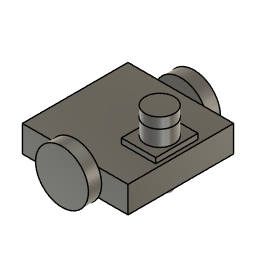
ros2bot (Autodesk Fusion 360 design; units mm, degrees)
Autodesk Fusion 360 part; units mm, degrees
sketch "Sketch1" plane through (0, 0, 0) normal (0, 0, 1) x (1, 0, 0)
  line L0 (-100, -100) -> (100, -100)
  line L1 (100, -100) -> (100, 100)
  line L2 (100, 100) -> (-100, 100)
  line L3 (-100, 100) -> (-100, -100)
  line L4 (-100, -100) -> (100, 100) construction
  line L5 (100, -100) -> (-100, 100) construction
  dimension "d1" = 200
  constraint horizontal L0
  constraint perpendicular L0 L1
  constraint parallel L0 L2
  constraint parallel L1 L3
  constraint coincident L4 origin
  constraint coincident L5 origin
  measures "d1" distance of L0.end L1.end
extrude "Extrude1" add sketch "Sketch1" along normal blind 50 makes body 1
sketch "Sketch2" plane through (0, -100, 0) normal (0, -1, 0) x (1, 0, 0)
  line L0 (-100, 0) -> (100, 0)
  line L1 (100, 0) -> (100, 50)
  line L2 (100, 50) -> (-100, 50)
  line L3 (-100, 50) -> (-100, 0)
  circle A0 centre (0, 25) radius 50
  dimension "d4" = 100
  measures "d4" diameter of A0
extrude "Extrude2" add sketch "Sketch2" along normal blind 25 separate body contours L0 L2 A0 | L0 A0 | L2 A0 makes body 2
mirror "Mirror1" about plane through (0, 0, 0) normal (0, 1, 0) of bodies 2 makes body 3
ref_plane "WorkPlane1" through (0, -116.4058, -25) normal (0, 0, -1) x (-1, 0, 0)
move_body "Move1" bodies 3 2 1 to x (1, 0, 0) y (0, 1, 0) z (0, 0, 1) at (0, 0, 25)
sketch "Sketch3" plane through (0, 0, 25) normal (0, 0, -1) x (1, 0, 0)
  line L0 (-100, 100) -> (-100, -100)
  line L1 (-100, -100) -> (100, -100)
  line L2 (100, -100) -> (100, 100)
  line L3 (100, 100) -> (-100, 100)
  circle A0 centre (75, 0) radius 10
  circle A1 centre (-70, 0) radius 10
  dimension "d10" = 20
  dimension "d11" = 20
  measures "d10" diameter of A0
  measures "d11" diameter of A1
extrude "Extrude3" add sketch "Sketch3" along normal blind 25 contours A0 | A1 bodies 1
fillet "Fillet1" radius 10 2 faces at (-70.8877, -1.6566, 0) (72.4279, -1.414, 0) on bodies 1
sketch "Sketch4" plane through (0, 0, 75) normal (0, 0, 1) x (-1, 0, 0)
  line L0 (100, -100) -> (100, 100)
  line L1 (100, 100) -> (-100, 100)
  line L2 (-100, 100) -> (-100, -100)
  line L3 (-100, -100) -> (100, -100)
  line L4 (-27.5, 40) -> (-92.5, 40)
  line L5 (-92.5, 40) -> (-92.5, -40)
  line L6 (-92.5, -40) -> (-27.5, -40)
  line L7 (-27.5, -40) -> (-27.5, 40)
  line L8 (-27.5, 40) -> (-92.5, -40) construction
  line L9 (-92.5, 40) -> (-27.5, -40) construction
  point P0 (-60, 0)
  dimension "d16" = 65
  dimension "d17" = 80
  constraint horizontal L4
  constraint perpendicular L4 L5
  constraint parallel L4 L6
  constraint parallel L5 L7
  constraint coincident L8 P0
  constraint coincident L9 P0
  measures "d16" distance of L5.end L6.end
  measures "d17" distance of L4.end L5.end
extrude "Extrude4" add sketch "Sketch4" along normal blind 10 contours L4 L5 L6 L7 bodies 1
sketch "Sketch5" plane through (0, 0, 85) normal (0, 0, 1) x (-1, 0, 0)
  line L0 (-27.5, -40) -> (-27.5, 40)
  line L1 (-27.5, 40) -> (-92.5, 40)
  line L2 (-92.5, 40) -> (-92.5, -40)
  line L3 (-92.5, -40) -> (-27.5, -40)
  circle A0 centre (-60, 0) radius 27.5
  dimension "d20" = 55
  measures "d20" diameter of A0
extrude "Extrude5" add sketch "Sketch5" along normal blind 30 contours A0 bodies 1
extrude "Extrude6" add 1 faces at (70.9837, -3.7731, 115) along direction (0, 0, 1) blind 20 separate body on bodies 1 makes body 4
copy_body "Body->Comp1" bodies 1 removing the originals makes body 5 in component "base_link"
copy_body "Body->Comp2" bodies 2 removing the originals makes body 6 in component "right_wheel"
copy_body "Body->Comp3" bodies 3 removing the originals makes body 7 in component "left_wheel"
copy_body "Body->Comp4" bodies 4 removing the originals makes body 8 in component "lidar"
component "base_link" placed x (1, 0, 0) y (0, 1, 0) z (0, 0, 1) at (0, 0, 0)
component "right_wheel" placed x (1, 0, 0) y (0, -1, 0) z (0, 0, -1) at (0, -225, 100)
component "left_wheel" placed x (1, 0, 0) y (0, -1, 0) z (0, 0, -1) at (0, 225, 100)
component "lidar" placed x (1, 0, 0) y (0, 1, 0) z (0, 0, 1) at (0, 0, 0)
